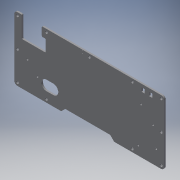
# Autodesk Inventor part: pcb
Saved by Autodesk Inventor 2019 (Build 230136000, 136)
## iProperties
Created: 2019-09-09
Part Number: pcb
Material: Generic
Document SubType Name: Modeling
Designer: jon
Density: 1 g/cm^3
Appearance: Default
Author: jon
Autodesk Inventor part; units mm, degrees
ref_plane "YZ Plane" through (0, 0, 0) normal (1, 0, 0) x (0, 1, 0)
ref_plane "XZ Plane" through (0, 0, 0) normal (0, 1, 0) x (-1, 0, 0)
ref_plane "XY Plane" through (0, 0, 0) normal (0, 0, 1) x (1, 0, 0)
sketch "Sketch1" plane through (0, 0, 0) normal (0, 0, 1) x (1, 0, 0)
  line L0 (150, 61) -> (150, 3)
  arc A0 (147, 0) -> (150, 3) centre (147, 3) ccw
  line L1 (147, 0) -> (100.4142, 0)
  arc A1 (99.7071, 0.2929) -> (100.4142, 0) centre (100.4142, 1) ccw
  line L2 (99.7071, 0.2929) -> (96.2929, 3.7071)
  arc A2 (96.2929, 3.7071) -> (95.5858, 4) centre (95.5858, 3) ccw
  line L3 (95.5858, 4) -> (51.4142, 4)
  arc A3 (51.4142, 4) -> (50.7071, 3.7071) centre (51.4142, 3) ccw
  line L4 (50.7071, 3.7071) -> (47.2929, 0.2929)
  arc A4 (46.5858, 0) -> (47.2929, 0.2929) centre (46.5858, 1) ccw
  line L5 (46.5858, 0) -> (3, 0)
  arc A5 (0, 3) -> (3, 0) centre (3, 3) ccw
  line L6 (0, 3) -> (0, 61)
  arc A6 (3, 64) -> (0, 61) centre (3, 61) ccw
  line L7 (3, 64) -> (6.5, 64)
  arc A7 (7.5, 63) -> (6.5, 64) centre (6.5, 63) ccw
  line L8 (7.5, 63) -> (7.5, 44)
  arc A8 (7.5, 44) -> (8.5, 43) centre (8.5, 44) ccw
  line L9 (8.5, 43) -> (30.5, 43)
  arc A9 (30.5, 43) -> (31.5, 44) centre (30.5, 44) ccw
  line L10 (31.5, 44) -> (31.5, 54)
  arc A10 (31.5, 54) -> (30.5, 55) centre (30.5, 54) ccw
  line L11 (30.5, 55) -> (28.5, 55)
  arc A11 (27.5, 56) -> (28.5, 55) centre (28.5, 56) ccw
  line L12 (27.5, 56) -> (27.5, 63)
  arc A12 (28.5, 64) -> (27.5, 63) centre (28.5, 63) ccw
  line L13 (28.5, 64) -> (147, 64)
  arc A13 (150, 61) -> (147, 64) centre (147, 61) ccw
  arc A14 (44, 15) -> (39, 20) centre (39, 15) ccw
  arc A15 (39, 10) -> (44, 15) centre (39, 15) ccw
  line L14 (39, 10) -> (32, 10)
  arc A16 (27, 15) -> (32, 10) centre (32, 15) ccw
  arc A17 (32, 20) -> (27, 15) centre (32, 15) ccw
  line L15 (32, 20) -> (39, 20)
  arc A18 (127.8, 60.9) -> (127.3, 60.4) centre (127.8, 60.4) ccw
  line L16 (127.3, 60.4) -> (127.3, 57.6)
  arc A19 (127.3, 57.6) -> (127.8, 57.1) centre (127.8, 57.6) ccw
  line L17 (127.8, 57.1) -> (130.2, 57.1)
  arc A20 (130.2, 57.1) -> (130.7, 57.6) centre (130.2, 57.6) ccw
  line L18 (127.8, 60.9) -> (130.2, 60.9)
  arc A21 (130.7, 60.4) -> (130.2, 60.9) centre (130.2, 60.4) ccw
  line L19 (130.7, 60.4) -> (130.7, 57.6)
  arc A22 (135.3, 60.9) -> (134.8, 60.4) centre (135.3, 60.4) ccw
  line L20 (134.8, 60.4) -> (134.8, 57.6)
  arc A23 (134.8, 57.6) -> (135.3, 57.1) centre (135.3, 57.6) ccw
  line L21 (135.3, 57.1) -> (137.7, 57.1)
  arc A24 (137.7, 57.1) -> (138.2, 57.6) centre (137.7, 57.6) ccw
  line L22 (135.3, 60.9) -> (137.7, 60.9)
  arc A25 (138.2, 60.4) -> (137.7, 60.9) centre (137.7, 60.4) ccw
  line L23 (138.2, 60.4) -> (138.2, 57.6)
  circle A26 centre (68, 60.85) radius 0.4
  circle A27 centre (68, 63.55) radius 0.4
  circle A28 centre (13, 28) radius 1
  circle A29 centre (23, 18) radius 1
  circle A30 centre (126.75, 46) radius 1
  circle A31 centre (138.75, 34) radius 1
  circle A32 centre (3, 61) radius 1.375
  circle A33 centre (32, 61) radius 1.375
  circle A34 centre (118, 61) radius 1.375
  circle A35 centre (147, 61) radius 1.375
  circle A36 centre (147, 3) radius 1.375
  circle A37 centre (118, 3) radius 1.375
  circle A38 centre (32, 3) radius 1.375
  circle A39 centre (3, 3) radius 1.375
  circle A40 centre (3, 32) radius 1.375
  circle A41 centre (75, 61) radius 1.375
  circle A42 centre (124, 9) radius 1
  circle A43 centre (142, 15) radius 1
  circle A44 centre (147, 32) radius 1.375
  point P0 (0, 0)
  constraints: 52 point on circle, 52 tangent, 48 end point, 45 centre point, 37 equal radius, 10 parallel, 10 perpendicular, 1 collinear
extrude "Extrusion1" add sketch "Sketch1" along normal blind 1.6
body "Solid1"
